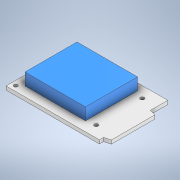
# Autodesk Inventor part: ProArduino
Saved by Autodesk Inventor 2022 (Build 260153000, 153)
## iProperties
Created: 2022-10-13
Part Number: ProArduino
Material: Generic
Document SubType Name: Modeling
Designer: richb366163
Density: 1 g/cm^3
Appearance: Default
Author: richb366163
Autodesk Inventor part; units mm, degrees
ref_plane "YZ Plane" through (0, 0, 0) normal (1, 0, 0) x (0, 1, 0)
ref_plane "XZ Plane" through (0, 0, 0) normal (0, 1, 0) x (-1, 0, 0)
ref_plane "XY Plane" through (0, 0, 0) normal (0, 0, 1) x (1, 0, 0)
sketch "Sketch1" plane through (0, 0, 0) normal (0, 1, 0) x (-1, 0, 0)
  line L0 (0, 0) -> (-78.3209, 0)
  line L1 (-78.3209, 0) -> (-78.3209, -57.3913)
  line L2 (-78.3209, -57.3913) -> (0, -57.3913)
  line L3 (0, -57.3913) -> (0, 0)
  line L4 (-78.3209, -3.4798) -> (-78.3209, -42.8625)
  line L5 (-83.4511, -4.9086) -> (-83.4511, -41.4338)
  line L6 (-78.3209, -3.4798) -> (-83.4511, -4.9086)
  line L7 (-83.4511, -41.4338) -> (-78.3209, -42.8625)
  line L8 (-78.3209, -57.3913) -> (-78.3209, -42.8625)
  dimension "d0" = 78.3209
  dimension "d1" = 57.3913
  dimension "d2" = 39.3827
  dimension "d3" = 36.5252
  dimension "d4" = 14.5288
  dimension "d5" = 5.1303
  constraints: 18 end point, 3 parallel, 2 vertical, 1 collinear, 1 equal length, 1 horizontal, 1 perpendicular, 1 point on line
  measures "d0" distance of L2.end L1.end
  measures "d1" distance of L1.end L0.end
  measures "d2" distance of L4.end L4.start
  measures "d3" distance of L5.start L5.end
  measures "d4" distance of L1.end L4.end
  measures "d5" horizontal distance of L4.end L5.end
extrude "Extrusion1" add sketch "Sketch1" along normal blind 3.048
sketch "Sketch2" plane through (0, 3.048, 0) normal (0, 1, 0) x (1, 0, 0)
  line L0 (78.3209, 57.3913) -> (0, 57.3913) projected
  line L1 (0, 57.3913) -> (2.3114, 57.3913)
  line L2 (2.3114, 57.3913) -> (2.3114, 54.6862)
  line L3 (2.3114, 54.6862) -> (0, 54.6862)
  line L4 (0, 54.6862) -> (0, 57.3913)
  line L5 (2.3114, 54.6862) -> (5.4864, 54.6862)
  line L6 (5.4864, 54.6862) -> (5.4864, 51.5874)
  line L7 (5.4864, 51.5874) -> (2.3114, 51.5874)
  line L8 (2.3114, 51.5874) -> (2.3114, 54.6862)
  circle A0 centre (3.8608, 53.1368) radius 1.5494
  line L9 (0, 57.3913) -> (0, 0) projected
  line L10 (0, 28.6957) -> (25.4, 28.6957)
  circle A1 centre (3.8608, 4.2545) radius 1.5494
  line L11 (0, 0) -> (78.3209, 0) projected
  line L12 (78.3209, 0) -> (67.8815, 0)
  line L13 (67.8815, 0) -> (67.8815, 57.3913)
  line L14 (67.8815, 57.3913) -> (78.3209, 57.3913)
  line L15 (78.3209, 57.3913) -> (78.3209, 0)
  line L16 (67.8815, 57.3913) -> (67.8815, 49.6443)
  line L17 (67.8815, 0) -> (67.8815, 7.747)
  line L18 (67.8815, 7.747) -> (64.7065, 7.747)
  line L19 (64.7065, 7.747) -> (64.7065, 10.922)
  line L20 (64.7065, 10.922) -> (67.8815, 10.922)
  line L21 (67.8815, 10.922) -> (67.8815, 7.747)
  line L22 (67.8815, 49.6443) -> (64.7065, 49.6443)
  line L23 (64.7065, 49.6443) -> (64.7065, 46.4693)
  line L24 (64.7065, 46.4693) -> (67.8815, 46.4693)
  line L25 (67.8815, 46.4693) -> (67.8815, 49.6443)
  circle A2 centre (66.294, 9.3345) radius 1.5875
  circle A3 centre (66.294, 48.0568) radius 1.5875
  dimension "d8" = 2.3114
  dimension "d9" = 2.7051
  dimension "d10" = 3.175
  dimension "d11" = 3.0988
  dimension "d12" = 10.4394
  dimension "d13" = 7.747
  dimension "d14" = 7.747
  dimension "d15" = 3.175
  dimension "d16" = 3.175
  dimension "d17" = 3.175
  dimension "d18" = 3.175
  constraints: 46 end point, 10 parallel, 6 horizontal, 5 perpendicular, 4 centre point, 3 point on line, 1 midpoint, 1 symmetric about line, 1 other
  measures "d8" distance of L2.end L3.end
  measures "d9" distance of L1.end L2.end
  measures "d10" distance of L6.end L7.end
  measures "d11" distance of L5.end L6.end
  measures "d12" distance of L13.end L14.end
  measures "d13" distance of L13.end L16.end
  measures "d14" distance of L12.end L17.end
  measures "d15" distance of L19.end L20.end
  measures "d16" distance of L18.end L19.end
  measures "d17" distance of L24.end L23.end
  measures "d18" distance of L23.end L22.end
extrude "Extrusion2" cut sketch "Sketch2" against normal blind 3.048 contours A3 | A0 | A2 | A1
sketch "Sketch3" plane through (0, 3.048, 0) normal (0, 1, 0) x (1, 0, 0)
  line L0 (7.9375, 51.5874) -> (58.7375, 51.5874)
  line L1 (58.7375, 51.5874) -> (58.7375, 7.9375)
  line L2 (58.7375, 7.9375) -> (7.9375, 7.9375)
  line L3 (7.9375, 7.9375) -> (7.9375, 51.5874)
  point P0 (0, 0)
  constraints: 8 end point, 2 parallel, 1 horizontal, 1 perpendicular
extrude "Extrusion3" add sketch "Sketch3" along normal blind 10.16
sketch "Sketch4" plane through (0, 0, 0) normal (0, -1, 0) x (1, 0, 0)
  line L0 (78.3209, -57.3913) -> (0, -57.3913) projected
  line L1 (0, 0) -> (78.3209, 0)
  line L2 (78.3209, 0) -> (78.3209, -57.3913)
  line L3 (78.3209, -57.3913) -> (0, -57.3913)
  line L4 (0, -57.3913) -> (0, 0)
  line L5 (0, 0) -> (78.3209, 0) projected
  line L6 (39.1604, 0) -> (39.1604, -57.3913)
  line L7 (78.3209, -28.6957) -> (0, -28.6957)
  line L8 (0, -57.3913) -> (0, 0) projected
  constraints: 12 end point, 4 midpoint, 2 parallel, 1 horizontal, 1 perpendicular
sketch "Sketch5" plane through (0, 0, 0) normal (0, -1, 0) x (1, 0, 0)
  line L0 (39.1604, 0) -> (39.1604, -57.3913) projected
  line L1 (78.3209, -28.6957) -> (0, -28.6957) projected
  circle A0 centre (3.8608, -53.1368) radius 1.5494 projected
  line L2 (39.1604, -28.6957) -> (3.8608, -28.6957)
  line L3 (3.8608, -28.6957) -> (3.8608, -53.1368)
  line L4 (3.8608, -53.1368) -> (39.1604, -53.1368)
  line L5 (39.1604, -53.1368) -> (39.1604, -28.6957)
  circle A1 centre (3.8608, -4.2545) radius 1.5494 projected
  line L6 (39.1604, -28.6957) -> (3.8608, -28.6957)
  line L7 (3.8608, -28.6957) -> (3.8608, -4.2545)
  line L8 (3.8608, -4.2545) -> (39.1604, -4.2545)
  line L9 (39.1604, -4.2545) -> (39.1604, -28.6957)
  circle A2 centre (66.294, -9.3345) radius 1.5875 projected
  line L10 (39.1604, -28.6957) -> (66.294, -28.6957)
  line L11 (66.294, -28.6957) -> (66.294, -9.3345)
  line L12 (66.294, -9.3345) -> (39.1604, -9.3345)
  line L13 (39.1604, -9.3345) -> (39.1604, -28.6957)
  circle A3 centre (66.294, -48.0568) radius 1.5875 projected
  line L14 (39.1604, -28.6957) -> (66.294, -28.6957)
  line L15 (66.294, -28.6957) -> (66.294, -48.0568)
  line L16 (66.294, -48.0568) -> (39.1604, -48.0568)
  line L17 (39.1604, -48.0568) -> (39.1604, -28.6957)
  point P0 (0, 0)
  dimension "d23" = 24.4412
  dimension "d24" = 24.4412
  dimension "d25" = 35.2996
  dimension "d26" = 35.2996
  dimension "d27" = 27.1335
  dimension "d28" = 27.1335
  dimension "d29" = 19.3611
  dimension "d30" = 19.3611
  constraints: 32 end point, 8 parallel, 4 horizontal, 4 perpendicular, 1 midpoint
  measures "d23" distance of L2.end L3.end
  measures "d24" distance of L6.end L7.end
  measures "d25" distance of L7.end L8.end
  measures "d26" distance of L3.end L4.end
  measures "d27" distance of L15.end L16.end
  measures "d28" distance of L11.end L12.end
  measures "d29" distance of L10.end L11.end
  measures "d30" distance of L14.end L15.end
body "Solid1"
